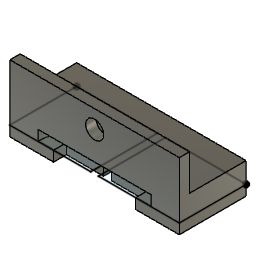
holder (Autodesk Fusion 360 design; units mm, degrees)
Autodesk Fusion 360 part; units mm, degrees
note: some values were not read from the file. Chosen so that the rebuilt part matches the saved one: where a step ends. Set by a fixed rule: which sketch regions a step uses.
sketch "スケッチ1" plane through (0, 0, 0) normal (0, 0, 1) x (1, 0, 0)
  line L0 (-16.5, 22) -> (16.5, 22)
  line L1 (16.5, 22) -> (16.5, 0)
  line L2 (16.5, 0) -> (-16.5, 0)
  line L3 (-16.5, 0) -> (-16.5, 22)
  dimension "d7" = 22
  dimension "d8" = 33
  constraint horizontal L0
  constraint vertical L1
  constraint horizontal L2
  constraint vertical L3
  constraint coincident origin L2
  constraint midpoint origin L2
  measures "d7" distance of L0.end L1.end
  measures "d8" distance of L0.start L0.end
extrude "押し出し1" add sketch "スケッチ1" along normal blind 2
sketch "スケッチ3" plane through (0, 0, 0) normal (0, 0, -1) x (1, 0, 0)
  line L0 (16.5, 0) -> (-16.5, 0)
  line L1 (-16.5, 0) -> (-16.5, -22)
  line L2 (-16.5, -22) -> (16.5, -22)
  line L3 (16.5, -22) -> (16.5, 0)
  arc A0 (-11, -9) -> (11, -9) centre (0, -9) ccw
  line L4 (16.5, -9) -> (-16.5, -9)
  dimension "d9" = 22
  dimension "d10" = 13
  constraint coincident L3 L4.start
  constraint coincident L1 L4.end
  constraint perpendicular L1 L4
  constraint coincident A0.centre L4
  measures "d9" diameter of A0
  measures "d10" distance of L2 A0.centre
extrude "押し出し2" add sketch "スケッチ3" along normal blind 2 contours L1 L2 L3 A0 L4
sketch "スケッチ4" plane through (0, 0, -2) normal (0, 0, -1) x (1, 0, 0)
  line L0 (-11, -9) -> (-16.5, -9)
  line L1 (-16.5, -9) -> (-16.5, -22)
  line L2 (-16.5, -22) -> (16.5, -22)
  line L3 (16.5, -22) -> (16.5, -9)
  line L4 (16.5, -9) -> (11, -9)
  arc A0 (-11, -9) -> (11, -9) centre (0, -9) ccw
  line L5 (16.5, -22) -> (0.75, -22)
  line L6 (0.75, -22) -> (0.75, -9)
  line L7 (0.75, -9) -> (16.5, -9)
  line L8 (16.5, -9) -> (16.5, -22)
  line L9 (-16.5, -22) -> (-0.75, -22)
  line L10 (-0.75, -22) -> (-0.75, -9)
  line L11 (-0.75, -9) -> (-16.5, -9)
  line L12 (-16.5, -9) -> (-16.5, -22)
  dimension "d13" = 1.5
  constraint horizontal L5
  constraint vertical L6
  constraint horizontal L7
  constraint vertical L8
  constraint coincident L2.end L3.start
  constraint horizontal L9
  constraint vertical L10
  constraint horizontal L11
  constraint vertical L12
  constraint coincident L1.end L2.start
  constraint equal L5 L9
  constraint equal L8 L12
  constraint equal L1 L12
  measures "d13" distance of L6 L10
extrude "押し出し3" add sketch "スケッチ4" along normal blind 2
sketch "スケッチ5" plane through (0, 0, 0) normal (0, 0, -1) x (1, 0, 0)
  line L0 (11, -9) -> (16.5, -9)
  line L1 (16.5, -9) -> (16.5, 0)
  line L2 (16.5, 0) -> (-16.5, 0)
  line L3 (-16.5, 0) -> (-16.5, -9)
  line L4 (-16.5, -9) -> (-11, -9)
  arc A0 (-11, -9) -> (11, -9) centre (0, -9) ccw
  line L5 (-3.75, 0) -> (3.75, 0)
  line L6 (3.75, 0) -> (3.75, -18)
  line L7 (3.75, -18) -> (-3.75, -18)
  line L8 (-3.75, -18) -> (-3.75, 0)
  line L9 (0, -1.75) -> (0, -22.5)
  line L10 (3.75, -7) -> (16.5, -7)
  line L11 (-3.75, -7) -> (-16.5, -7)
  dimension "d17" = 7.5
  dimension "d18" = 11
  dimension "d19" = 11
  constraint horizontal L5
  constraint vertical L6
  constraint horizontal L7
  constraint vertical L8
  constraint coincident L2 L5.start
  constraint symmetric L6 L8 L9
  constraint coincident L6 L10.start
  constraint perpendicular L6 L10
  constraint coincident L1 L10.end
  constraint coincident L8 L11.start
  constraint coincident L3 L11.end
  constraint perpendicular L3 L11
  measures "d17" distance of L5.start L5.end
  measures "d18" distance of L6.end L10.start
  measures "d19" distance of L7.end L11.start
sketch "スケッチ9" plane through (0, 9, 0) normal (0, -1, 0) x (1, 0, 0)
  line L0 (-11, 0) -> (-16.5, 0)
  line L1 (-16.5, 0) -> (-16.5, -4)
  line L2 (-16.5, -4) -> (-0.75, -4)
  line L3 (-0.75, -4) -> (-0.75, -2)
  line L4 (-0.75, -2) -> (-11, -2)
  line L5 (-11, -2) -> (-11, 0)
  line L6 (-8, -2) -> (8, -2)
  line L7 (8, -2) -> (8, -4)
  line L8 (8, -4) -> (-8, -4)
  line L9 (-8, -4) -> (-8, -2)
  line L10 (16.5, -4) -> (0.75, -4)
  dimension "d37" = 16
  dimension "d38" = 8
  constraint horizontal L6
  constraint vertical L7
  constraint horizontal L8
  constraint vertical L9
  constraint coincident L4 L6.start
  constraint collinear L8 L10
  measures "d37" distance of L7.end L8.end
  measures "d38" distance of origin L7
extrude "押し出し7" cut sketch "スケッチ9" against normal blind 2.5 contours L2 L3 L4 L6 L8 L9 | L3 L6 L7 L8 L10
sketch "スケッチ11" plane through (0, 22, 0) normal (0, 1, 0) x (-1, 0, 0)
  line L0 (16.5, -4) -> (16.5, 2)
  line L1 (16.5, 2) -> (-16.5, 2)
  line L2 (-16.5, 2) -> (-16.5, -4)
  line L3 (-16.5, -4) -> (16.5, -4)
  line L4 (16.5, 2) -> (-13.5, 2)
  line L5 (-13.5, 2) -> (-13.5, 12)
  line L6 (-13.5, 12) -> (16.5, 12)
  line L7 (16.5, 12) -> (16.5, 2)
  dimension "d49" = 10
  constraint horizontal L4
  constraint vertical L5
  constraint horizontal L6
  constraint vertical L7
  constraint coincident L0.end L1.start
  measures "d49" distance of L0.end L6.end
ref_plane "作業平面1" through (0, 11, -1) normal (0, 1, 0) x (-1, 0, 0)
sketch "スケッチ13" plane through (0, 11, -1) normal (0, 1, 0) x (1, 0, 0)
  line L0 (16.5, -10) -> (-16.5, -10)
  line L1 (-16.5, -10) -> (-16.5, -3)
  line L2 (-16.5, -3) -> (16.5, -3)
  line L3 (16.5, -3) -> (16.5, -10)
  line L4 (16.5, 3) -> (16.5, -3)
  line L5 (-16.5, 3) -> (-16.5, -3)
  circle A0 centre (0, -6.5) radius 1.75
  dimension "d53" = 7
  dimension "d54" = 3.5
  dimension "d58" = 3.5
  constraint horizontal L0
  constraint vertical L1
  constraint horizontal L2
  constraint vertical L3
  constraint collinear L3 L4
  constraint collinear L1 L5
  constraint coincident L2 L1.end
  measures "d53" distance of L0.end L1.end
  measures "d54" diameter of A0
  measures "d58" distance of L2 A0.centre
extrude "押し出し11" add sketch "スケッチ13" against normal blind 2
sketch "スケッチ14" plane through (-16.5, 0, 0) normal (-1, 0, 0) x (0, -1, 0)
  line L0 (-9, 0) -> (0, 0)
  line L1 (0, 0) -> (0, 2)
  line L2 (0, 2) -> (-9, 2)
  line L3 (-9, 2) -> (-9, 9)
  line L4 (-9, 9) -> (-11, 9)
  line L5 (-11, 9) -> (-11, 2)
  line L6 (-11, 2) -> (-22, 2)
  line L7 (-22, 2) -> (-22, -4)
  line L8 (-22, -4) -> (-9, -4)
  line L9 (-9, -4) -> (-9, 0)
  line L10 (0, 2) -> (-9, 2)
  line L11 (-9, 2) -> (-9, 0)
  line L12 (-9, 0) -> (0, 0)
  line L13 (0, 0) -> (0, 2)
  constraint horizontal L10
  constraint vertical L11
  constraint horizontal L12
  constraint vertical L13
  constraint coincident L0.start L9.end
  constraint coincident L1.end L2.start
extrude "押し出し12" cut sketch "スケッチ14" along normal up to far side of body 1 contours L0 L1 L2 L10 L11 L12 L13
